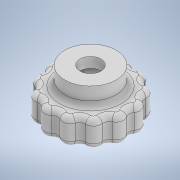
# Autodesk Inventor part: Idom KNOB
Saved by Autodesk Inventor 2020 (Build 240168000, 168)
## iProperties
Created: 2022-05-04
Part Number: Idom KNOB
Material: Genérico
Document SubType Name: Modeling
Designer: aarco
Density: 1 g/cm^3
Appearance: Valor por defecto
Author: aarco
Autodesk Inventor part; units mm, degrees
ref_plane "YZ Plane" through (0, 0, 0) normal (1, 0, 0) x (0, 1, 0)
ref_plane "XZ Plane" through (0, 0, 0) normal (0, 1, 0) x (-1, 0, 0)
ref_plane "XY Plane" through (0, 0, 0) normal (0, 0, 1) x (1, 0, 0)
sketch "Boceto1" plane through (0, 0, 0) normal (0, 1, 0) x (-1, 0, 0)
  circle A0 centre (0, 0) radius 17.5
  dimension "d0" = 35
  constraints: 1 centre point, 1 coincident
  measures "d0" diameter of A0
extrude "Extrusión1" add sketch "Boceto1" along normal blind 10
sketch "Boceto2" plane through (0, 10, 0) normal (0, 1, 0) x (1, 0, 0)
  circle A0 centre (0, 0) radius 10
  dimension "d3" = 20
  constraints: 1 centre point, 1 coincident
  measures "d3" diameter of A0
extrude "Extrusión2" add sketch "Boceto2" along normal blind 7
sketch "Boceto3" plane through (0, 0, 0) normal (0, -1, 0) x (1, 0, 0)
  circle A0 centre (0, 0) radius 4.1
  dimension "d6" = 8.2
  constraints: 1 centre point, 1 coincident
  measures "d6" diameter of A0
extrude "Extrusión3" cut sketch "Boceto3" against normal through all
sketch "Boceto4" plane through (0, 0, 0) normal (0, -1, 0) x (1, 0, 0)
  circle A0 centre (0, 0) radius 4.1 projected
  line L0 (-6.365, 3.6748) -> (0, 7.3497)
  line L1 (0, 7.3497) -> (6.365, 3.6748)
  line L2 (6.365, 3.6748) -> (6.365, -3.6748)
  line L3 (6.365, -3.6748) -> (0, -7.3497)
  line L4 (0, -7.3497) -> (-6.365, -3.6748)
  line L5 (-6.365, -3.6748) -> (-6.365, 3.6748)
  dimension "d9" = 12.73
  constraints: 12 end point, 1 coincident, 1 vertical, 13 other
  measures "d9" distance between parallel lines of L2 L5
extrude "Extrusión4" cut sketch "Boceto4" against normal blind 13 contours A0 | L0 L1 L2 L3 L4 L5
sketch "Boceto5" plane through (0, 0, 0) normal (0, -1, 0) x (1, 0, 0)
  circle A0 centre (0, 0) radius 17.5 projected
  circle A1 centre (17.5, 0) radius 2.5
  line L0 (0, 0) -> (17.5, 0)
  dimension "d12" = 5
  constraints: 2 end point, 1 centre point, 1 horizontal, 1 horizontal alignment, 1 other
  measures "d12" diameter of A1
extrude "Extrusión5" cut sketch "Boceto5" against normal through all contours L0 A1 A0 | A0 A1 | A0 A1 L0 picked at (18.2366, 0.6547)
pattern_circular "Patrón circular1" count 13 over 360 about axis through (0, 0, 0) along (0, 1, 0) of "Extrusión5"
fillet "Empalme1" radius 3 26 edges at (17.3214, 5, -2.4936) (17.3214, 5, 2.4936) (14.1785, 5, -10.2577) (16.4962, 5, -5.8417) (11.8919, 5, -12.8387) (7.7875, 5, -15.6718) (-0.3876, 5, -17.4957) (4.5633, 5, -16.8946) (-8.4738, 5, -15.3116) (-3.8107, 5, -17.0801) (-14.6188, 5, -9.6197) (-11.3117, 5, -13.3527) (-17.4149, 5, -1.7241) (-16.2213, 5, -6.5664) (16.4962, 5, 5.8417) (14.1785, 5, 10.2577) (11.8919, 5, 12.8387) (7.7875, 5, 15.6718) (4.5633, 5, 16.8946) (-0.3876, 5, 17.4957) (-3.8107, 5, 17.0801) (-8.4738, 5, 15.3116) (-11.3117, 5, 13.3527) (-14.6188, 5, 9.6197) (-17.4149, 5, 1.7241) (-16.2213, 5, 6.5664)
fillet "Empalme2" radius 2 52 edges at (15, 0, 0) (15.9495, 0, -3.9312) (13.2818, 0, -6.9708) (12.2957, 0, -10.893) (8.521, 0, -12.3448) (5.825, 0, -15.3594) (1.8081, 0, -14.8906) (-1.98, 0, -16.3071) (-5.3191, 0, -14.0252) (-9.3315, 0, -13.519) (-11.2277, 0, -9.9468) (-14.5453, 0, -7.6339) (-14.5641, 0, -3.5897) (-16.4269, 0, 0) (-14.5641, 0, 3.5897) (-14.5453, 0, 7.6339) (-11.2277, 0, 9.9468) (-9.3315, 0, 13.519) (-5.3191, 0, 14.0252) (-1.98, 0, 16.3071) (1.8081, 0, 14.8906) (5.825, 0, 15.3594) (8.521, 0, 12.3448) (12.2957, 0, 10.893) (13.2818, 0, 6.9708) (15.9495, 0, 3.9312) (5.825, 10, 15.3594) (8.521, 10, 12.3448) (12.2957, 10, 10.893) (13.2818, 10, 6.9708) (15.9495, 10, 3.9312) (15, 10, 0) (15.9495, 10, -3.9312) (13.2818, 10, -6.9708) (12.2957, 10, -10.893) (8.521, 10, -12.3448) (5.825, 10, -15.3594) (1.8081, 10, -14.8906) (-1.98, 10, -16.3071) (-5.3191, 10, -14.0252) (-9.3315, 10, -13.519) (-11.2277, 10, -9.9468) (-14.5453, 10, -7.6339) (-14.5641, 10, -3.5897) (-16.4269, 10, 0) (-14.5641, 10, 3.5897) (-14.5453, 10, 7.6339) (-11.2277, 10, 9.9468) (-9.3315, 10, 13.519) (-5.3191, 10, 14.0252) (-1.98, 10, 16.3071) (1.8081, 10, 14.8906)
fillet "Empalme3" radius 2 1 edges at (-10, 10, 0)
fillet "Empalme4" radius 1 6 edges at (3.1825, 0, 5.5123) (-3.1825, 0, 5.5123) (-6.365, 0, 0) (-3.1825, 0, -5.5123) (3.1825, 0, -5.5123) (6.365, 0, 0)
